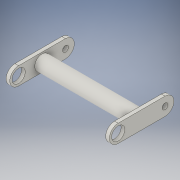
# Autodesk Inventor part: toggle
Saved by Autodesk Inventor 2017 (Build 210142000, 142)
## iProperties
Created: 2017-01-16
Part Number: toggle
Material: Steel, Wrought
Document SubType Name: Modeling
Designer: mmarkle
Density: 7.85 g/cm^3
Appearance: Steel
Mass: 766.745 g
Surface Area: 426.832 cm^2
Volume: 97.6745 cm^3
Author: mmarkle
Autodesk Inventor part; units mm, degrees
ref_plane "YZ Plane" through (0, 0, 0) normal (1, 0, 0) x (0, 1, 0)
ref_plane "XZ Plane" through (0, 0, 0) normal (0, 1, 0) x (-1, 0, 0)
sketch "Sketch1" plane through (0, 0, 0) normal (1, 0, 0) x (0, 1, 0)
  line L0 (0, -50.8) -> (0, 50.8) construction
  line L1 (19.05, -50.8) -> (19.05, 50.8)
  line L2 (-19.05, 50.8) -> (-19.05, -50.8)
  arc A0 (-19.05, -50.8) -> (19.05, -50.8) centre (0, -50.8) ccw
  arc A1 (19.05, 50.8) -> (-19.05, 50.8) centre (0, 50.8) ccw
  circle A2 centre (0, 50.8) radius 14.2875
  circle A3 centre (0, -50.8) radius 6.35
  point P0 (0, 0)
  dimension "d0" = 50.8
  dimension "d1" = 38.1
  dimension "d2" = 28.575
  dimension "d12" = 12.7
  constraints: 8 end point, 4 centre point, 4 point on circle, 4 tangent, 2 coincident, 1 midpoint, 1 parallel, 1 vertical
  measures "d0" distance of point (0, 0) L0.end
  measures "d1" diameter of A1
  measures "d2" diameter of A2
  measures "d12" diameter of A3
extrude "Extrusion1" add sketch "Sketch1" along normal blind 7.9375
sketch "Sketch2" plane through (7.9375, 0, 0) normal (1, 0, 0) x (0, 0, -1)
  circle A0 centre (0, 0) radius 12.7
  circle A1 centre (0, 0) radius 15.875
  dimension "d5" = 25.4
  dimension "d6" = 31.75
  constraints: 2 centre point, 2 coincident
  measures "d5" diameter of A0
  measures "d6" diameter of A1
extrude "Extrusion2" add sketch "Sketch2" along normal blind 207.9625
ref_plane "Work Plane1" through (215.9, 0, 0) normal (1, 0, 0) x (0, 0, -1)
sketch "Sketch3" plane through (215.9, 0, 0) normal (1, 0, 0) x (0, 0, -1)
  arc A0 (-50.8, 19.05) -> (-50.8, -19.05) centre (-50.8, 0) ccw projected
  circle A1 centre (-50.8, 0) radius 14.2875 projected
  line L0 (50.8, 19.05) -> (-50.8, 19.05) projected
  arc A2 (50.8, -19.05) -> (50.8, 19.05) centre (50.8, 0) ccw projected
  line L1 (-50.8, -19.05) -> (50.8, -19.05) projected
  circle A3 centre (50.8, 0) radius 6.35 projected
  point P0 (0, 0)
  dimension "d13" = 101.6
  measures "d13" distance of A0.centre A2.centre
extrude "Extrusion3" add sketch "Sketch3" along normal blind 7.9375
body "Solid1"
